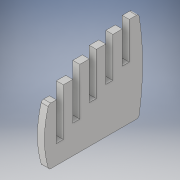
# Autodesk Inventor part: Head Frame
Saved by Autodesk Inventor 2019 (Build 230136000, 136)
## iProperties
Created: 2020-02-12
Part Number: Head Frame
Material: Generic
Document SubType Name: Modeling
Designer: student
Density: 1 g/cm^3
Appearance: Default
Author: student
Autodesk Inventor part; units mm, degrees
ref_plane "YZ Plane" through (0, 0, 0) normal (1, 0, 0) x (0, 1, 0)
ref_plane "XZ Plane" through (0, 0, 0) normal (0, 1, 0) x (-1, 0, 0)
ref_plane "XY Plane" through (0, 0, 0) normal (0, 0, 1) x (1, 0, 0)
sketch "Sketch1" plane through (0, 0, 0) normal (1, 0, 0) x (0, 1, 0)
  line L0 (0, 0) -> (60.325, 0) construction
  line L1 (60.325, 0) -> (60.325, -60.325) construction
  line L2 (60.325, -60.325) -> (0, -60.325) construction
  line L3 (0, -60.325) -> (0, 0) construction
  line L4 (0, 0) -> (0, -60.325)
  line L5 (0, -60.325) -> (60.325, -60.325) construction
  line L6 (38.1, -5.08) -> (12.7, -5.08)
  line L7 (12.7, -5.08) -> (12.7, -9.779)
  line L8 (12.7, -9.779) -> (44.45, -9.779)
  line L9 (44.45, -9.779) -> (44.45, -16.129)
  line L10 (44.45, -16.129) -> (19.05, -16.129)
  line L11 (19.05, -16.129) -> (19.05, -20.828)
  line L12 (38.1, -5.08) -> (38.1, 0)
  line L13 (0, 0) -> (38.1, 0) construction
  line L14 (19.05, -20.828) -> (50.8, -20.828)
  line L15 (50.8, -20.828) -> (50.8, -27.178)
  line L16 (50.8, -27.178) -> (25.4, -27.178)
  line L17 (25.4, -27.178) -> (25.4, -31.877)
  line L18 (25.4, -31.877) -> (53.975, -31.877)
  line L19 (53.975, -31.877) -> (53.975, -38.227)
  line L20 (60.325, -60.325) -> (60.325, -53.975)
  line L21 (60.325, -53.975) -> (35.56, -53.975)
  line L22 (35.56, -53.975) -> (35.56, -49.276)
  line L23 (35.56, -49.276) -> (57.15, -49.276)
  line L24 (57.15, -49.276) -> (57.15, -42.926)
  line L25 (57.15, -42.926) -> (30.48, -42.926)
  line L26 (30.48, -42.926) -> (30.48, -38.227)
  line L27 (30.48, -38.227) -> (53.975, -38.227)
  arc A0 (38.1, 0) -> (0, 0) centre (19.05, -60.5751) ccw
  arc A1 (0, -60.325) -> (60.325, -60.325) centre (30.1625, 114.8979) ccw
  dimension "d0" = 60.325
  dimension "d1" = 60.325
  dimension "d2" = 4.699
  dimension "d3" = 5.08
  dimension "d5" = 6.35
  dimension "d6" = 6.35
  dimension "d7" = 4.699
  dimension "d8" = 12.7
  dimension "d9" = 25.4
  dimension "d10" = 25.4
  dimension "d11" = 6.35
  dimension "d12" = 4.699
  dimension "d13" = 6.35
  dimension "d14" = 25.4
  dimension "d15" = 6.35
  dimension "d18" = 4.699
  dimension "d19" = 4.699
  dimension "d22" = 6.35
  dimension "d28" = 5.08
  dimension "d35" = 63.5
  dimension "d36" = 177.8
  dimension "d39" = 6.35
  dimension "d40" = 3.175
  dimension "d42" = 5.08
  dimension "d43" = 3.175
  constraints: 56 end point, 14 perpendicular, 4 equal length, 4 point on circle, 4 vertical, 3 horizontal, 2 centre point, 2 point on line
  measures "d0" distance of L2.end L0.start
  measures "d1" distance of L1.end L2.end
  measures "d2" distance between parallel lines of L8 L6
  measures "d3" distance between parallel lines of L0 L6
  measures "d5" distance of L8.end L9.end
  measures "d6" distance from line of L10.end L7
  measures "d7" distance of L10.end L11.end
  measures "d8" distance between parallel lines of L3 L7
  measures "d9" distance of L6.start L6.end
  measures "d10" distance of L9.end L10.end
  measures "d11" distance of L14.end L15.end
  measures "d12" distance of L16.end L17.end
  measures "d13" distance between parallel lines of L11 L17
  measures "d14" distance of L15.end L16.end
  measures "d15" distance of L18.end L19.end
  measures "d18" distance of L25.end L26.end
  measures "d19" distance of L21.end L22.end
  measures "d22" distance of L23.end L24.end
  measures "d28" distance between parallel lines of L26 L22
  measures "d35" radius of A0
  measures "d36" radius of A1
  measures "d39" distance of L1.end L20.end
  measures "d40" distance between parallel lines of L20 L24
  measures "d42" distance between parallel lines of L17 L26
  measures "d43" distance between parallel lines of L15 L19
extrude "Extrusion1" add sketch "Sketch1" against normal blind 4.699
fillet "Fillet1" radius 1.7145 4 edges at (-2.3495, 38.1, 0) (-2.3495, 0, 0) (-2.3495, 0, -60.325) (-2.3495, 60.325, -60.325)
equation "\"d2\" = thick"
equation "\"d6\" = 0.5 * d8"
equation "\"d7\" = thick"
equation "\"d12\" = thick"
equation "\"d13\" = d6"
equation "\"d18\" = thick"
equation "\"d19\" = thick"
equation "\"thick\" = 4.699"
body "Solid1"
